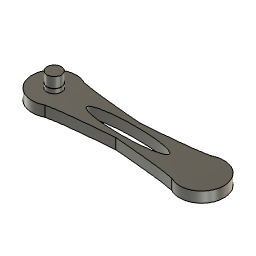
Second Arm (Autodesk Fusion 360 design; units mm, degrees)
Autodesk Fusion 360 part; units mm, degrees
note: some values were not read from the file. Set by a fixed rule: which sketch regions a step uses.
sketch "Sketch1" plane through (0, 0, 0) normal (0, 0, 1) x (1, 0, 0)
  circle A0 centre (0, 0) radius 11.1125
  circle A1 centre (0, 0) radius 15
  line L0 (0, 0) -> (100, 0)
  circle A2 centre (100, 0) radius 11.1125
  circle A3 centre (100, 0) radius 15
  line L1 (0, 0) -> (50, 0)
  line L2 (50, 0) -> (50, 43.1808)
  spline S0 degree 5 poles (7.0229, 13.2544) (7.3818, 13.1855) (8.0878, 13.0509) (9.1117, 12.8585) (10.4065, 12.6211) (11.91, 12.3559) (13.3078, 12.1213) (14.6194, 11.9144) (15.8799, 11.7303) (17.1392, 11.5615) (18.4486, 11.4002) (19.8513, 11.2391) (21.369, 11.0732) (22.998, 10.9002) (24.7193, 10.7202) (26.5058, 10.5344) (28.3301, 10.3446) (30.1733, 10.1529) (32.0282, 9.9607) (33.895, 9.7694) (35.7793, 9.5798) (37.6894, 9.3928) (39.6334, 9.2089) (41.6168, 9.0285) (43.6429, 8.8518) (45.7133, 8.6789) (47.4056, 8.5436) (48.695, 8.4438) (49.5635, 8.378) (50, 8.3454) knots 0 0 0 0 0 0 0.04 0.08 0.12 0.16 0.2 0.24 0.28 0.32 0.36 0.4 0.44 0.48 0.52 0.56 0.6 0.64 0.68 0.72 0.76 0.8 0.84 0.88 0.92 0.96 1 1 1 1 1 1
  spline S1 degree 5 poles (92.9771, 13.2544) (92.6182, 13.1855) (91.9122, 13.0509) (90.8883, 12.8585) (89.5935, 12.6211) (88.09, 12.3559) (86.6922, 12.1213) (85.3806, 11.9144) (84.1201, 11.7303) (82.8608, 11.5615) (81.5514, 11.4002) (80.1487, 11.2391) (78.631, 11.0732) (77.002, 10.9002) (75.2807, 10.7202) (73.4942, 10.5344) (71.6699, 10.3446) (69.8267, 10.1529) (67.9718, 9.9607) (66.105, 9.7694) (64.2207, 9.5798) (62.3106, 9.3928) (60.3666, 9.2089) (58.3832, 9.0285) (56.3571, 8.8518) (54.2867, 8.6789) (52.5944, 8.5436) (51.305, 8.4438) (50.4365, 8.378) (50, 8.3454) knots 0 0 0 0 0 0 0.04 0.08 0.12 0.16 0.2 0.24 0.28 0.32 0.36 0.4 0.44 0.48 0.52 0.56 0.6 0.64 0.68 0.72 0.76 0.8 0.84 0.88 0.92 0.96 1 1 1 1 1 1
  line L3 (1.9267, 14.2328) -> (12.1192, 12.2759)
  line L4 (45.3075, 8.6968) -> (54.6925, 7.994)
  line L5 (98.0733, 14.2328) -> (87.8808, 12.2759)
  line L6 (54.6925, 8.6968) -> (45.3075, 7.994)
  spline S2 degree 5 poles (7.0229, -13.2544) (7.3818, -13.1855) (8.0878, -13.0509) (9.1117, -12.8585) (10.4065, -12.6211) (11.91, -12.3559) (13.3078, -12.1213) (14.6194, -11.9144) (15.8799, -11.7303) (17.1392, -11.5615) (18.4486, -11.4002) (19.8513, -11.2391) (21.369, -11.0732) (22.998, -10.9002) (24.7193, -10.7202) (26.5058, -10.5344) (28.3301, -10.3446) (30.1733, -10.1529) (32.0282, -9.9607) (33.895, -9.7694) (35.7793, -9.5798) (37.6894, -9.3928) (39.6334, -9.2089) (41.6168, -9.0285) (43.6429, -8.8518) (45.7133, -8.6789) (47.4056, -8.5436) (48.695, -8.4438) (49.5635, -8.378) (50, -8.3454) knots 0 0 0 0 0 0 0.04 0.08 0.12 0.16 0.2 0.24 0.28 0.32 0.36 0.4 0.44 0.48 0.52 0.56 0.6 0.64 0.68 0.72 0.76 0.8 0.84 0.88 0.92 0.96 1 1 1 1 1 1
  line L7 (1.9267, -14.2328) -> (12.1192, -12.2759)
  line L8 (45.3075, -8.6968) -> (54.6925, -7.994)
  spline S3 degree 5 poles (92.9771, -13.2544) (92.6182, -13.1855) (91.9122, -13.0509) (90.8883, -12.8585) (89.5935, -12.6211) (88.09, -12.3559) (86.6922, -12.1213) (85.3806, -11.9144) (84.1201, -11.7303) (82.8608, -11.5615) (81.5514, -11.4002) (80.1487, -11.2391) (78.631, -11.0732) (77.002, -10.9002) (75.2807, -10.7202) (73.4942, -10.5344) (71.6699, -10.3446) (69.8267, -10.1529) (67.9718, -9.9607) (66.105, -9.7694) (64.2207, -9.5798) (62.3106, -9.3928) (60.3666, -9.2089) (58.3832, -9.0285) (56.3571, -8.8518) (54.2867, -8.6789) (52.5944, -8.5436) (51.305, -8.4438) (50.4365, -8.378) (50, -8.3454) knots 0 0 0 0 0 0 0.04 0.08 0.12 0.16 0.2 0.24 0.28 0.32 0.36 0.4 0.44 0.48 0.52 0.56 0.6 0.64 0.68 0.72 0.76 0.8 0.84 0.88 0.92 0.96 1 1 1 1 1 1
  line L9 (98.0733, -14.2328) -> (87.8808, -12.2759)
  line L10 (54.6925, -8.6968) -> (45.3075, -7.994)
  ellipse E0 centre (50, 0) end of major axis (22.0571, 0) minor radius 4.9455
  line L11 (77.9429, 0) -> (22.0571, 0) construction
  line L12 (50, 4.9455) -> (50, -4.9455) construction
  point P0 (14.1243, 11.9944)
  point P1 (19.3372, 11.2994)
  point P2 (27.5042, 10.4305)
  point P3 (37.7564, 9.388)
  point P4 (85.8757, 11.9944)
  point P5 (80.6628, 11.2994)
  point P6 (72.4958, 10.4305)
  point P7 (62.2436, 9.388)
  point P8 (14.1243, -11.9944)
  point P9 (19.3372, -11.2994)
  point P10 (27.5042, -10.4305)
  point P11 (37.7564, -9.388)
  point P12 (85.8757, -11.9944)
  point P13 (80.6628, -11.2994)
  point P14 (72.4958, -10.4305)
  point P15 (62.2436, -9.388)
  dimension "d1" = 22.225
  dimension "d2" = 30
  dimension "d3" = 100
  dimension "d4" = 22.225
  dimension "d5" = 30
  dimension "d6" = 50
  constraint coincident A0.centre A1.centre
  constraint concentric A0 A1
  constraint horizontal L0
  constraint coincident L0.end A2.centre
  constraint concentric A2 A3
  constraint parallel L0 L1
  constraint perpendicular L1 L2
  constraint coincident A1 S0.start
  constraint coincident L2 S0.end
  constraint midpoint S0.start L3
  constraint midpoint S0.end L4
  constraint symmetric L2 S0.start S1.start
  constraint symmetric L2 P0 P4
  constraint symmetric L2 P1 P5
  constraint symmetric L2 P2 P6
  constraint symmetric L2 P3 P7
  constraint symmetric L2 S0.end S1.end
  constraint symmetric L2 L3.start L5.start
  constraint symmetric L2 L3.end L5.end
  constraint symmetric L2 L4.start L6.start
  constraint symmetric L2 L4.end L6.end
  constraint symmetric L0 S0.start S2.start
  constraint symmetric L0 P0 P8
  constraint symmetric L0 P1 P9
  constraint symmetric L0 P2 P10
  constraint symmetric L0 P3 P11
  constraint symmetric L0 S0.end S2.end
  constraint symmetric L0 S1.start S3.start
  constraint symmetric L0 P4 P12
  constraint symmetric L0 P5 P13
  constraint symmetric L0 P6 P14
  constraint symmetric L0 P7 P15
  constraint symmetric L0 L3.start L7.start
  constraint symmetric L0 L3.end L7.end
  constraint symmetric L0 L4.start L8.start
  constraint symmetric L0 L4.end L8.end
  constraint symmetric L0 L5.start L9.start
  constraint symmetric L0 L5.end L9.end
  constraint symmetric L0 L6.start L10.start
  constraint symmetric L0 L6.end L10.end
  constraint coincident E0 L11.start
  constraint coincident E0 L11.end
  constraint coincident E0 L12.start
  constraint coincident E0 L12.end
  constraint coincident L1.end L2.start
  constraint perpendicular L2 L11
  measures "d1" diameter of A0
  measures "d2" diameter of A1
  measures "d3" distance of A0.centre L0.end
  measures "d4" diameter of A2
  measures "d5" diameter of A3
  measures "d6" distance of A0.centre L1.end
extrude "Extrude2" add sketch "Sketch1" along normal blind 7.142 contours A0 | A1 | A1 L0 A3 L1 S2 S3 E0 | A1 L0 L1 L2 S0 E0 | L0 A3 L2 S1 E0 | A3 | A2
sketch "Sketch2" plane through (0, 0, 7.142) normal (0, 0, 1) x (-1, 0, 0)
  arc A0 (-7.0229, -13.2544) -> (-7.0229, 13.2544) centre (0, 0) ccw
  arc A1 (-92.9771, 13.2544) -> (-92.9771, -13.2544) centre (-100, 0) ccw
  circle A2 centre (0, 0) radius 5
  circle A3 centre (0, 0) radius 4.875
  spline S0 degree 5 poles (-50, -8.3454) (-49.5635, -8.378) (-48.695, -8.4438) (-47.4056, -8.5436) (-45.7133, -8.6789) (-43.6429, -8.8518) (-41.6168, -9.0285) (-39.6334, -9.2089) (-37.6894, -9.3928) (-35.7793, -9.5798) (-33.895, -9.7694) (-32.0282, -9.9607) (-30.1733, -10.1529) (-28.3301, -10.3446) (-26.5058, -10.5344) (-24.7193, -10.7202) (-22.998, -10.9002) (-21.369, -11.0732) (-19.8513, -11.2391) (-18.4486, -11.4002) (-17.1392, -11.5615) (-15.8799, -11.7303) (-14.6194, -11.9144) (-13.3078, -12.1213) (-11.91, -12.3559) (-10.4065, -12.6211) (-9.1117, -12.8585) (-8.0878, -13.0509) (-7.3818, -13.1855) (-7.0229, -13.2544) knots -1 -1 -1 -1 -1 -1 -0.96 -0.92 -0.88 -0.84 -0.8 -0.76 -0.72 -0.68 -0.64 -0.6 -0.56 -0.52 -0.48 -0.44 -0.4 -0.36 -0.32 -0.28 -0.24 -0.2 -0.16 -0.12 -0.08 -0.04 0 0 0 0 0 0
  spline S1 degree 5 poles (-7.0229, 13.2544) (-7.3818, 13.1855) (-8.0878, 13.0509) (-9.1117, 12.8585) (-10.4065, 12.6211) (-11.91, 12.3559) (-13.3078, 12.1213) (-14.6194, 11.9144) (-15.8799, 11.7303) (-17.1392, 11.5615) (-18.4486, 11.4002) (-19.8513, 11.2391) (-21.369, 11.0732) (-22.998, 10.9002) (-24.7193, 10.7202) (-26.5058, 10.5344) (-28.3301, 10.3446) (-30.1733, 10.1529) (-32.0282, 9.9607) (-33.895, 9.7694) (-35.7793, 9.5798) (-37.6894, 9.3928) (-39.6334, 9.2089) (-41.6168, 9.0285) (-43.6429, 8.8518) (-45.7133, 8.6789) (-47.4056, 8.5436) (-48.695, 8.4438) (-49.5635, 8.378) (-50, 8.3454) knots 0 0 0 0 0 0 0.04 0.08 0.12 0.16 0.2 0.24 0.28 0.32 0.36 0.4 0.44 0.48 0.52 0.56 0.6 0.64 0.68 0.72 0.76 0.8 0.84 0.88 0.92 0.96 1 1 1 1 1 1
  spline S2 degree 5 poles (-50, 8.3454) (-50.4365, 8.378) (-51.305, 8.4438) (-52.5944, 8.5436) (-54.2867, 8.6789) (-56.3571, 8.8518) (-58.3832, 9.0285) (-60.3666, 9.2089) (-62.3106, 9.3928) (-64.2207, 9.5798) (-66.105, 9.7694) (-67.9718, 9.9607) (-69.8267, 10.1529) (-71.6699, 10.3446) (-73.4942, 10.5344) (-75.2807, 10.7202) (-77.002, 10.9002) (-78.631, 11.0732) (-80.1487, 11.2391) (-81.5514, 11.4002) (-82.8608, 11.5615) (-84.1201, 11.7303) (-85.3806, 11.9144) (-86.6922, 12.1213) (-88.09, 12.3559) (-89.5935, 12.6211) (-90.8883, 12.8585) (-91.9122, 13.0509) (-92.6182, 13.1855) (-92.9771, 13.2544) knots -1 -1 -1 -1 -1 -1 -0.96 -0.92 -0.88 -0.84 -0.8 -0.76 -0.72 -0.68 -0.64 -0.6 -0.56 -0.52 -0.48 -0.44 -0.4 -0.36 -0.32 -0.28 -0.24 -0.2 -0.16 -0.12 -0.08 -0.04 0 0 0 0 0 0
  spline S3 degree 5 poles (-92.9771, -13.2544) (-92.6182, -13.1855) (-91.9122, -13.0509) (-90.8883, -12.8585) (-89.5935, -12.6211) (-88.09, -12.3559) (-86.6922, -12.1213) (-85.3806, -11.9144) (-84.1201, -11.7303) (-82.8608, -11.5615) (-81.5514, -11.4002) (-80.1487, -11.2391) (-78.631, -11.0732) (-77.002, -10.9002) (-75.2807, -10.7202) (-73.4942, -10.5344) (-71.6699, -10.3446) (-69.8267, -10.1529) (-67.9718, -9.9607) (-66.105, -9.7694) (-64.2207, -9.5798) (-62.3106, -9.3928) (-60.3666, -9.2089) (-58.3832, -9.0285) (-56.3571, -8.8518) (-54.2867, -8.6789) (-52.5944, -8.5436) (-51.305, -8.4438) (-50.4365, -8.378) (-50, -8.3454) knots 0 0 0 0 0 0 0.04 0.08 0.12 0.16 0.2 0.24 0.28 0.32 0.36 0.4 0.44 0.48 0.52 0.56 0.6 0.64 0.68 0.72 0.76 0.8 0.84 0.88 0.92 0.96 1 1 1 1 1 1
  ellipse E0 centre (-50, 0) end of major axis (-22.0571, 0) minor radius 4.9455
  dimension "d13" = 10
  dimension "d14" = 9.75
  constraint coincident A0.centre A2.centre
  measures "d13" diameter of A2
  measures "d14" diameter of A3
extrude "Extrude3" add sketch "Sketch2" along normal blind 3 contours A2
extrude "Extrude4" add 1 faces at (-1.2886, 0.6786, 7.142) along direction (0, 0, 1) blind 10
sketch "Sketch3" plane through (0, 0, 17.142) normal (0, 0, 1) x (-1, 0, 0)
  circle A0 centre (0, 0) radius 4.875
  circle A1 centre (0.0174, -4.875) radius 0.2855
  circle A2 centre (4.875, 0.0174) radius 0.2855
  circle A3 centre (-0.0174, 4.875) radius 0.2855
  circle A4 centre (-4.875, -0.0174) radius 0.2855
  dimension "d19" = 0.571
  dimension "d21" = 360
  constraint coincident A0 A1.centre
  measures "d19" diameter of A1
